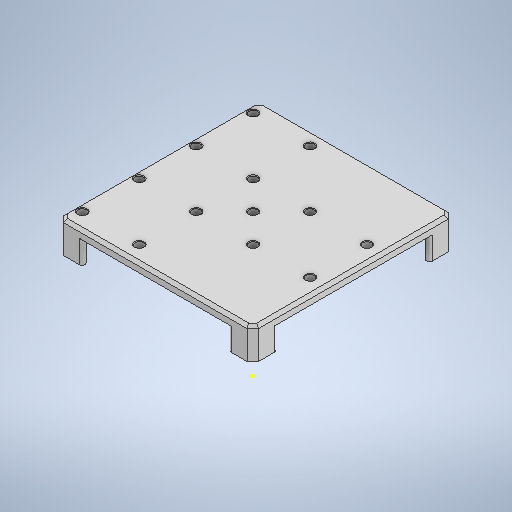
# Autodesk Inventor part: Repick
Saved by Autodesk Inventor 2025 (Build 290162000, 162)
## iProperties
Created: 2026-07-17
Part Number: Repick
Material: Generic
Document SubType Name: Sheet Metal
Designer: MSI
Density: 1 g/cm^3
Sheet Metal Rule: Default_mm
Appearance: Default
Author: MSI
Autodesk Inventor part; units mm, degrees
ref_plane "YZ Plane" through (0, 0, 0) normal (1, 0, 0) x (0, 1, 0)
ref_plane "XZ Plane" through (0, 0, 0) normal (0, 1, 0) x (-1, 0, 0)
ref_plane "XY Plane" through (0, 0, 0) normal (0, 0, 1) x (1, 0, 0)
sketch "Sketch1" plane through (0, 0, 0) normal (0, 1, 0) x (-1, 0, 0)
  circle A0 centre (80, -20) radius 1.5
  circle A1 centre (80, -40) radius 1.5
  circle A2 centre (80, -60) radius 1.5
  circle A3 centre (80, -80) radius 1.5
  circle A4 centre (60, -80) radius 1.5
  circle A5 centre (60, -60) radius 1.5
  circle A6 centre (60, -40) radius 1.5
  circle A7 centre (60, -20) radius 1.5
  circle A8 centre (20, -60) radius 1.5
  circle A9 centre (20, -40) radius 1.5
  circle A10 centre (40, -60) radius 1.5
  circle A11 centre (40, -40) radius 1.5
  circle A12 centre (50, -50) radius 1.5
  line L0 (82.9894, -14.3145) -> (14.4573, -14.3145)
  line L1 (14.4573, -14.3145) -> (14.4573, -84.9883)
  line L2 (14.4573, -84.9883) -> (82.9894, -84.9883)
  line L3 (82.9894, -84.9883) -> (82.9894, -14.3145)
  point P0 (0, 0)
  dimension "d4" = 3
  dimension "d5" = 3
  dimension "d6" = 3
  dimension "d7" = 3
  dimension "d8" = 3
  dimension "d9" = 3
  dimension "d10" = 3
  dimension "d11" = 3
  dimension "d13" = 3
  dimension "d14" = 3
  dimension "d15" = 3
  dimension "d16" = 3
  dimension "d17" = 60
  dimension "d20" = 3
  constraints: 13 centre point, 8 end point, 2 parallel, 1 horizontal, 1 perpendicular
  measures "d4" diameter of A0
  measures "d5" diameter of A1
  measures "d6" diameter of A2
  measures "d7" diameter of A3
  measures "d8" diameter of A4
  measures "d9" diameter of A5
  measures "d10" diameter of A6
  measures "d11" diameter of A7
  measures "d13" diameter of A8
  measures "d14" diameter of A9
  measures "d15" diameter of A10
  measures "d16" diameter of A11
  measures "d17" distance of A3.centre A0.centre
  measures "d20" diameter of A12
extrude "Extrusion1" add sketch "Sketch1" along normal blind 3
chamfer "Chamfer1" distance 2 angle 45 4 edges at (-14.4573, 1.5, -14.3145) (-14.4573, 1.5, -84.9883) (-82.9894, 1.5, -84.9883) (-82.9894, 1.5, -14.3145)
sketch "Sketch2" plane through (0, 0, 0) normal (0, -1, 0) x (1, 0, 0)
  line L0 (-14.4573, -16.3145) -> (-14.4573, -82.9883) projected
  line L1 (-14.4573, -82.9883) -> (-14.4573, -74.9883)
  line L2 (-16.4573, -84.9883) -> (-80.9894, -84.9883) projected
  line L3 (-16.4573, -84.9883) -> (-24.4573, -84.9883)
  line L4 (-24.4573, -84.9883) -> (-14.4573, -74.9883)
  line L5 (-16.4573, -84.9883) -> (-14.4573, -82.9883) projected
  line L6 (-16.4573, -84.9883) -> (-14.4573, -82.9883)
  line L7 (-80.9894, -84.9883) -> (-72.9894, -84.9883)
  line L8 (-82.9894, -82.9883) -> (-82.9894, -16.3145) projected
  line L9 (-80.9894, -84.9883) -> (-82.9894, -82.9883)
  line L10 (-82.9894, -82.9883) -> (-82.9894, -74.9883)
  line L11 (-82.9894, -74.9883) -> (-72.9894, -84.9883)
  line L12 (-80.9894, -14.3145) -> (-16.4573, -14.3145) projected
  line L13 (-16.4573, -14.3145) -> (-24.4573, -14.3145)
  line L14 (-16.4573, -14.3145) -> (-14.4573, -16.3145)
  line L15 (-14.4573, -16.3145) -> (-14.4573, -24.3145)
  line L16 (-14.4573, -24.3145) -> (-24.4573, -14.3145)
  line L17 (-82.9894, -16.3145) -> (-82.9894, -24.3145)
  line L18 (-82.9894, -16.3145) -> (-80.9894, -14.3145)
  line L19 (-80.9894, -14.3145) -> (-72.9894, -14.3145)
  line L20 (-72.9894, -14.3145) -> (-82.9894, -24.3145)
  point P0 (0, 0)
  dimension "d26" = 8
  dimension "d27" = 8
  dimension "d28" = 8
  dimension "d29" = 8
  dimension "d30" = 8
  dimension "d31" = 8
  dimension "d32" = 8
  dimension "d33" = 8
  constraints: 32 end point, 8 point on line, 1 collinear
  measures "d26" distance of L0.end L1.end
  measures "d27" distance of L2.start L3.end
  measures "d28" distance of L2.end L7.end
  measures "d29" distance of L8.start L10.end
  measures "d30" distance of L12.end L13.end
  measures "d31" distance of L0.start L15.end
  measures "d32" distance of L8.end L17.end
  measures "d33" distance of L12.start L19.end
extrude "Extrusion2" add sketch "Sketch2" along normal blind 8 contours L0 L16 L12 L14 | L0 L5 L2 L4 | L20 L8 L18 L12 | L2 L9 L8 L11
extrude "Extrusion3" cut sketch "Sketch1" against normal blind 3 contours A0 | A3
fillet "Fillet1" radius 1 1 edges at (-82.9894, -4, -24.3145)
fillet "Fillet2" radius 1 7 edges at (-72.9894, -4, -14.3145) (-14.4573, -4, -24.3145) (-14.4573, -4, -74.9883) (-24.4573, -4, -84.9883) (-72.9894, -4, -84.9883) (-24.4573, -4, -14.3145) (-82.9894, -4, -74.9883)
chamfer "Chamfer2" distance 0.2 angle 45 13 edges at (-78.5, 3, -80) (-58.5, 3, -80) (-58.5, 3, -60) (-78.5, 3, -60) (-38.5, 3, -60) (-18.5, 3, -60) (-18.5, 3, -40) (-38.5, 3, -40) (-48.5, 3, -50) (-58.5, 3, -40) (-58.5, 3, -20) (-78.5, 3, -40) (-78.5, 3, -20)
chamfer "Chamfer3" distance 1 angle 45 8 edges at (-48.7233, 3, -14.3145) (-14.4573, 3, -49.6514) (-48.7233, 3, -84.9883) (-82.9894, 3, -49.6514) (-81.9894, 3, -83.9883) (-15.4573, 3, -83.9883) (-15.4573, 3, -15.3145) (-81.9894, 3, -15.3145)
sketch "Sketch4" plane through (0, 3, 0) normal (0, 1, 0) x (1, 0, 0)
  point P0 (0, 0)
equation "\"BendRadius\" = Thickness"
equation "\"BendReliefWidth\" = Thickness"
equation "\"BendReliefDepth\" = 0.5 * Thickness"
equation "\"CornerReliefSize\" = 4 * Thickness"
equation "\"MinimumRemnant\" = 2 * Thickness"
equation "\"TransitionRadius\" = BendRadius"
equation "\"JacobiRadiusSize\" = BendRadius"
equation "\"GapSize\" = Thickness"
equation "\"Thickness\" = 0.5"
body "Solid1"
